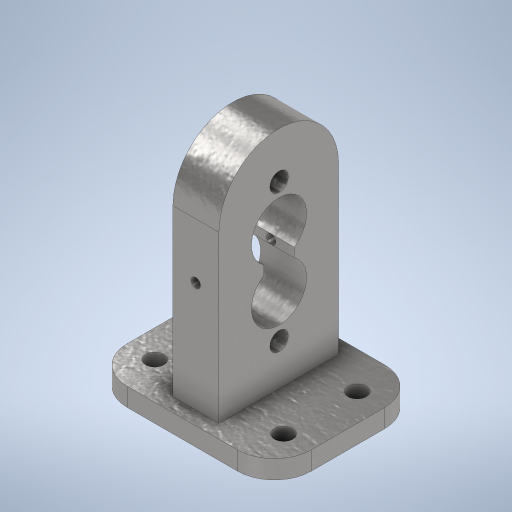
# Autodesk Inventor part: grave
Saved by Autodesk Inventor 2024 (Build 280153000, 153)
## iProperties
Created: 2024-02-08
Part Number: grave
Material: Stahl, galvanisiert
Document SubType Name: Modeling
Designer: ffogue
Density: 7.85 g/cm^3
Appearance: Galvanisiert
Author: ffogue
Autodesk Inventor part; units mm, degrees
ref_plane "XY Plane" through (0, 0, 0) normal (0, 0, 1) x (1, 0, 0)
sketch "Skizze1" plane through (0, 0, 0) normal (0, 0, 1) x (1, 0, 0)
  line L0 (0, 8) -> (10, 8)
  line L1 (10, 8) -> (10, 0)
  line L2 (10, 0) -> (0, 0)
  line L3 (0, 0) -> (0, 8)
  dimension "d0" = 8
  dimension "d1" = 10
  constraints: 8 end point, 2 parallel, 1 coincident, 1 horizontal, 1 perpendicular
  measures "d0" distance between parallel lines of L2 L0
  measures "d1" distance between parallel lines of L1 L3
extrude "Extrusion1" add sketch "Skizze1" along normal mid plane 1
ref_plane "Arbeitsebene2" through (5, 0, 0) normal (1, 0, 0) x (0, 1, 0)
sketch "Skizze3" plane through (5, 0, 0) normal (1, 0, 0) x (0, 1, 0)
  line L0 (8, 0.5) -> (0, 0.5) projected
  line L1 (0.7344, 0.5) -> (7.2344, 0.5)
  line L2 (7.2344, 0.5) -> (7.2344, 9.5)
  line L3 (0.7344, 9.5) -> (0.7344, 0.5)
  arc A0 (7.2344, 9.5) -> (0.7344, 9.5) centre (3.9844, 9.5) ccw
  line L4 (0, -0.5) -> (8, -0.5) projected
  point P0 (0, 0)
  point P1 (3.9844, -0.5)
  dimension "d5" = 6.5
  dimension "d6" = 10
  constraints: 6 end point, 2 point on circle, 2 tangent, 1 centre point, 1 horizontal, 1 parallel, 1 perpendicular, 1 point on line, 1 vertical alignment, 2 other
  measures "d5" distance between parallel lines of L2 L3
extrude "Extrusion2" add sketch "Skizze3" along normal mid plane 2.5
sketch "Skizze4" plane through (6.25, 0, 0) normal (1, 0, 0) x (0, 0, -1)
  line L0 (-6.75, 3.1708) -> (-6.25, 3.1708)
  line L1 (-6.75, 4.8292) -> (-6.25, 4.8292)
  arc A0 (-6.75, 4.8292) -> (-6.75, 3.1708) centre (-8, 4) ccw
  arc A1 (-6.25, 3.1708) -> (-6.25, 4.8292) centre (-5, 4) ccw
  line L2 (-0.5, 0) -> (-0.5, 8) projected
  point P0 (0, 0)
  point P1 (-0.5, 4)
  dimension "d9" = 1.5
  dimension "d10" = 0.5
  dimension "d11" = 4.5
  dimension "d12" = 3
  constraints: 4 end point, 4 point on circle, 2 centre point, 2 horizontal, 2 horizontal alignment, 2 vertical alignment, 1 equal radius, 1 midpoint
  measures "d9" radius of A0
  measures "d10" distance of L0.start L0.end
  measures "d11" distance from line of L2 A1.centre
  measures "d12" distance of A0.centre A1.centre
extrude "Extrusion3" cut sketch "Skizze4" against normal blind 2.5
sketch "Skizze5" plane through (6.25, 0, 0) normal (1, 0, 0) x (0, 0, -1)
  arc A0 (-6.25, 3.1708) -> (-6.25, 4.8292) centre (-5, 4) ccw projected
  point P0 (0, 0)
  point P1 (-2.75, 4)
  point P2 (-3.5, 4)
  point P3 (-3.5, 4)
  dimension "d15" = 0.75
  constraints: 2 point on circle, 1 horizontal alignment
  measures "d15" distance of point (-3.5, 4) point (-2.75, 4)
hole "Bohrung1" at (6.25, 4, 2.75) direction (-1, 0, 0) diameter 1 end through all
sketch "Skizze6" plane through (6.25, 0, 0) normal (1, 0, 0) x (0, 0, -1)
  arc A0 (-6.75, 4.8292) -> (-6.75, 3.1708) centre (-8, 4) ccw projected
  point P0 (0, 0)
  point P1 (-10.25, 4)
  point P2 (-9.5, 4)
  point P3 (-9.5, 4)
  dimension "d23" = 0.75
  constraints: 2 point on circle, 1 horizontal alignment
  measures "d23" distance of point (-9.5, 4) point (-10.25, 4)
hole "Bohrung2" at (6.25, 4, 10.25) direction (-1, 0, 0) diameter 1 end through all
ref_plane "Arbeitsebene3" through (0, 4, 0) normal (0, 1, 0) x (-1, 0, 0)
sketch "Skizze7" plane through (0, 4, 0) normal (0, 1, 0) x (-1, 0, 0)
  circle A0 centre (-5, 6.4964) radius 0.2536
  line L0 (-6.25, 6.75) -> (-3.75, 6.75) projected
  point P0 (0, 0)
  point P1 (-5, 6.75)
  dimension "d32" = 0.5072
  constraints: 1 centre point, 1 midpoint, 1 tangent, 1 vertical alignment
  measures "d32" diameter of A0
extrude "Extrusion4" cut sketch "Skizze7" along normal through all both and the other way through all
fillet "Rundung1" radius 2 4 edges at (10, 8, 0) (10, 0, 0) (0, 8, 0) (0, 0, 0)
sketch "Skizze8" plane through (0, 0, 0.5) normal (0, 0, 1) x (1, 0, 0)
  line L0 (10, 2) -> (10, 6) projected
  line L1 (10, 4) -> (0, 4) construction
  line L2 (2, 0) -> (8, 0) projected
  line L3 (5, 0) -> (5, 8) construction
  line L4 (2, 8) -> (8, 8) projected
  point P0 (0, 0)
  point P1 (8.5, 2)
  point P2 (1.5, 2)
  point P3 (1.5, 6)
  point P4 (8.5, 6)
  dimension "d36" = 7
  dimension "d37" = 4
  constraints: 4 end point, 3 midpoint, 3 symmetric about line, 1 horizontal
  measures "d36" distance of point (1.5, 2) point (8.5, 2)
  measures "d37" distance of point (1.5, 6) point (1.5, 2)
hole "Bohrung3" at (8.5, 2, 0.5) at (1.5, 2, 0.5) at (1.5, 6, 0.5) at (8.5, 6, 0.5) direction (0, 0, -1) diameter 1 end through all
